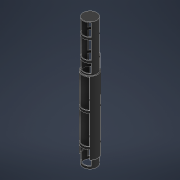
# Autodesk Inventor part: Test_Electronics_ Housing
Saved by Autodesk Inventor 2022 (Build 260153000, 153)
## iProperties
Created: 2024-05-09
Part Number: Test_Electronics_ Housing
Material: Generic
Document SubType Name: Modeling
Designer: jo_ki
Density: 1 g/cm^3
Appearance: Rubber - Black
Author: jo_ki
Autodesk Inventor part; units mm, degrees
ref_plane "YZ Plane" through (0, 0, 0) normal (1, 0, 0) x (0, 1, 0)
ref_plane "XZ Plane" through (0, 0, 0) normal (0, 1, 0) x (-1, 0, 0)
sketch "Sketch1" plane through (0, 0, 0) normal (0, 0, 1) x (1, 0, 0)
  line L0 (0, -222.05) -> (0, 149.3) projected
  line L1 (0, 0) -> (14, 0)
  line L2 (14, 0) -> (14, 96.25)
  line L3 (14, 96.25) -> (0, 96.25)
  line L4 (0, 96.25) -> (0, 0)
  line L5 (0, 0) -> (16, 0)
  line L6 (16, 0) -> (16, -150)
  line L7 (16, -150) -> (0, -150)
  line L8 (0, -150) -> (0, 0)
  line L9 (0, -150) -> (14, -150)
  line L10 (14, -150) -> (14, -169)
  line L11 (14, -169) -> (0, -169)
  line L12 (0, -169) -> (0, -150)
  line L13 (12.5, 94.75) -> (0, 94.75)
  line L14 (0, 94.75) -> (0, -1.5)
  line L15 (0, -1.5) -> (12.5, -1.5)
  line L16 (12.5, -1.5) -> (12.5, 94.75)
  line L17 (12.5, -167.5) -> (0, -167.5)
  line L18 (0, -167.5) -> (0, -148.5)
  line L19 (0, -148.5) -> (12.5, -148.5)
  line L20 (12.5, -148.5) -> (12.5, -167.5)
  line L21 (0, -1.5) -> (14.5, -1.5)
  line L22 (14.5, -1.5) -> (14.5, -148.5)
  line L23 (14.5, -148.5) -> (0, -148.5)
  line L24 (0, -148.5) -> (0, -1.5)
  line L25 (12.5, -167.5) -> (14, -167.5)
  point P0 (0, 96.25)
  point P1 (0, -169)
  point P2 (14, 0)
  point P3 (0, 94.75)
  point P4 (12.5, -1.5)
  point P5 (0, -167.5)
  dimension "d0" = 28
  dimension "d1" = 96.25
  dimension "d3" = 150
  dimension "d4" = 19
  dimension "d7" = 32
  dimension "d8" = 28
  dimension "d13" = 1.5
  dimension "d14" = 1.5
  dimension "d15" = 1.5
  dimension "d16" = 1.5
  dimension "d17" = 1.5
  dimension "d18" = 1.5
  constraints: 50 end point, 12 parallel, 7 perpendicular, 6 horizontal, 5 point on line, 2 collinear
  measures "d0" diameter of L2 L0
  measures "d1" distance of L1.end L2.end
  measures "d3" distance of L5.end L6.end
  measures "d4" distance of L9.end L10.end
  measures "d7" diameter of L6 L0
  measures "d8" diameter of L10 L0
  measures "d13" distance between parallel lines of L6 L22
  measures "d14" distance between parallel lines of L16 L2
  measures "d15" distance between parallel lines of L5 L21
  measures "d16" distance between parallel lines of L7 L23
  measures "d17" distance between parallel lines of L11 L17
  measures "d18" distance between parallel lines of L3 L13
revolve "Revolution1" add sketch "Sketch1" angle 360 about axis through (0, -10, 0) along (0, 1, 0) contours L20 L7 L10 L25 | L20 L23 L22 L21 L16 L1 L5 L6 L7 | L0 L3 L2 L1 L16 L13
sketch "Sketch2" plane through (0, 0, 0) normal (0, 1, 0) x (-1, 0, 0)
  circle A0 centre (0, 0) radius 16 projected
  line L0 (6, -12.6491) -> (6, -14.8324)
  circle A1 centre (0, 0) radius 16 projected
  line L1 (-6, -12.6491) -> (-6, -14.8324)
  line L2 (0, -22.4) -> (0, 22.4) projected
  circle A2 centre (0, 0) radius 14 projected
  point P0 (0, 16)
  point P1 (0, -16)
  dimension "d9" = 12
  constraints: 4 end point, 1 parallel, 1 point on circle, 1 vertical, 5 other
  measures "d9" distance between parallel lines of L1 L0
extrude "Extrusion1" [suppressed]
sketch "Sketch3" plane through (0, 0, 0) normal (0, 0, 1) x (1, 0, 0)
  line L0 (11, 94.75) -> (-11, 94.75)
  line L1 (-11, 94.75) -> (-11, -167.5)
  line L2 (-11, -167.5) -> (11, -167.5)
  line L3 (11, -167.5) -> (11, 94.75)
  line L4 (12.5, -167.5) -> (12.5, -148.5) projected
  line L5 (-12.5, -167.5) -> (-12.5, -148.5) projected
  line L6 (0, -219.95) -> (0, 147.2) projected
  line L7 (-12.5, -167.5) -> (12.5, -167.5) projected
  line L8 (-12.5, 94.75) -> (12.5, 94.75) projected
  line L9 (11, -131.5) -> (-11, -131.5)
  line L10 (-11, -131.5) -> (-11, -126.5)
  line L11 (-11, -126.5) -> (11, -126.5)
  line L12 (11, -126.5) -> (11, -131.5)
  line L13 (11, -66.5) -> (-11, -66.5)
  line L14 (-11, -66.5) -> (-11, -61.5)
  line L15 (-11, -61.5) -> (11, -61.5)
  line L16 (11, -61.5) -> (11, -66.5)
  line L17 (-12.5, -1.5) -> (-12.5, 94.75) projected
  line L18 (11, -1.5) -> (-12.5, -1.5)
  line L19 (-12.5, -1.5) -> (-12.5, 3.5)
  line L20 (-12.5, 3.5) -> (11, 3.5)
  line L21 (11, 3.5) -> (11, -1.5)
  line L22 (11, 63.5) -> (-11, 63.5)
  line L23 (-11, 63.5) -> (-11, 68.5)
  line L24 (-11, 68.5) -> (11, 68.5)
  line L25 (11, 68.5) -> (11, 63.5)
  line L26 (0, -126.5) -> (0, -66.5)
  line L27 (0, -61.5) -> (0, -1.5)
  line L28 (0, 3.5) -> (0, 63.5)
  line L29 (-12.5, -1.5) -> (12.5, -1.5) projected
  line L30 (-16, 0) -> (16, 0) projected
  line L31 (-16, -150) -> (16, -150) projected
  line L32 (-6, 0) -> (6, 0)
  line L33 (6, 0) -> (6, 27)
  line L34 (6, 27) -> (-6, 27)
  line L35 (-6, 27) -> (-6, 0)
  line L36 (11, 22) -> (-11, 22)
  line L37 (-11, 22) -> (-11, 27)
  line L38 (-11, 27) -> (11, 27)
  line L39 (11, 27) -> (11, 22)
  line L40 (-6, 22) -> (11, 22)
  line L41 (-12.5, -162.5) -> (12.5, -162.5)
  line L42 (12.5, -162.5) -> (12.5, -167.5)
  line L43 (12.5, -167.5) -> (-12.5, -167.5)
  line L44 (-12.5, -167.5) -> (-12.5, -162.5)
  point P0 (0, 0)
  point P1 (-11, -131.5)
  point P2 (-11, -66.5)
  point P3 (11, -126.5)
  point P4 (-11, -1.5)
  point P5 (11, -61.5)
  point P6 (-11, 63.5)
  point P7 (-11, 3.5)
  point P8 (11, 3.5)
  point P9 (11, 68.5)
  point P10 (-11, 22)
  point P11 (11, 27)
  point P12 (6, 22)
  point P13 (6, 3.5)
  point P14 (-6, 3.5)
  point P15 (-11, -162.5)
  point P16 (11, -162.5)
  dimension "d19" = 1.5
  dimension "d22" = 5
  dimension "d23" = 5
  dimension "d24" = 5
  dimension "d25" = 5
  dimension "d26" = 60
  dimension "d27" = 5
  dimension "d32" = 5
  constraints: 72 end point, 18 point on line, 16 parallel, 8 horizontal, 8 perpendicular, 7 collinear, 4 midpoint, 1 other
  measures "d19" distance between parallel lines of L3 L4
  measures "d22" distance between parallel lines of L11 L9
  measures "d23" distance between parallel lines of L13 L15
  measures "d24" distance between parallel lines of L18 L20
  measures "d25" distance between parallel lines of L22 L24
  measures "d26" distance of L27.start L27.end
  measures "d27" distance between parallel lines of L36 L38
  measures "d32" distance between parallel lines of L7 L41
extrude "Extrusion2" cut sketch "Sketch3" along normal through all both and the other way through all contours L3 L24 L6 L0 | L6 L24 L1 L0 | L3 L38 L34 L6 L22 | L6 L34 L38 L1 L22 | L3 L20 L33 L36 | L1 L36 L35 L20 | L36 L33 L20 L6 | L6 L20 L35 L36 | L18 L6 L15 L1 | L3 L15 L6 L18 | L13 L6 L11 L1 | L3 L11 L6 L13 | L9 L6 L31 L1 | L3 L31 L6 L9 | L31 L6 L41 L1 | L3 L41 L6 L31
sketch "Sketch4" plane through (0, 0, 0) normal (0, 1, 0) x (-1, 0, 0)
  circle A0 centre (0, 0) radius 16 projected
  circle A1 centre (0, 0) radius 12.5 projected
  line L0 (6, -10.9659) -> (6, -14.8324)
  line L1 (-6, -14.8324) -> (-6, -10.9659)
  line L2 (0, -22.4) -> (0, 22.4) projected
  dimension "d33" = 12
  constraints: 4 end point, 4 point on circle, 1 parallel, 1 vertical, 1 other
  measures "d33" distance between parallel lines of L1 L0
extrude "Extrusion3" add sketch "Sketch4" along normal blind 27 and the other way blind 5 contours A0 L2 A1 L0 | A0 L1 A1 L2 picked at (3.409, -13.2047) picked at (-3.409, -13.2047)
ref_plane "Work Plane1" through (0, -75, -16) normal (0, 0, 1) x (1, 0, 0)
sketch "Sketch5" plane through (0, -75, -16) normal (0, 0, 1) x (1, 0, 0)
  line L0 (-6, 73.5) -> (-11, 73.5) projected
  line L1 (-11, 73.5) -> (-11, 13.5) projected
  line L2 (-11, 13.5) -> (11, 13.5) projected
  line L3 (11, 13.5) -> (11, 73.5) projected
  line L4 (11, 73.5) -> (6, 73.5) projected
  line L5 (6, 70) -> (6, 73.5) projected
  line L6 (-6, 70) -> (6, 70) projected
  line L7 (-6, 73.5) -> (-6, 70) projected
  line L8 (6, 75) -> (-6, 75) projected
  line L9 (-6, 102) -> (-6, 75) projected
  line L10 (6, 102) -> (-6, 102) projected
  line L11 (6, 75) -> (6, 102) projected
  line L12 (11, -56.5) -> (11, -75) projected
  line L13 (11, -75) -> (11, -75) projected
  line L14 (11, -75) -> (11, -56.5) projected
  line L15 (11, -56.5) -> (-11, -56.5) projected
  line L16 (-11, -56.5) -> (-11, -75) projected
  line L17 (-11, -75) -> (-11, -75) projected
  line L18 (-11, -75) -> (-11, -56.5) projected
  line L19 (-11, -56.5) -> (11, -56.5) projected
  line L20 (-11, 73.5) -> (11, 73.5) projected
  line L21 (11, 73.5) -> (11, 13.5) projected
  line L22 (11, 13.5) -> (-11, 13.5) projected
  line L23 (-11, 13.5) -> (-11, 73.5) projected
  line L24 (-11, 8.5) -> (11, 8.5) projected
  line L25 (11, 8.5) -> (11, -51.5) projected
  line L26 (11, -51.5) -> (-11, -51.5) projected
  line L27 (-11, -51.5) -> (-11, 8.5) projected
  line L28 (11, 8.5) -> (-11, 8.5) projected
  line L29 (-11, 8.5) -> (-11, -51.5) projected
  line L30 (-11, -51.5) -> (11, -51.5) projected
  line L31 (11, -51.5) -> (11, 8.5) projected
  line L32 (-6, 70) -> (6, 70) projected
  line L33 (-6, 70) -> (-6, 102)
  line L34 (-6, 102) -> (-6, 75) projected
  line L35 (-6, 86) -> (6, 86)
  line L36 (0, -145.25) -> (0, 224) projected
  point P0 (0, 75)
  point P1 (0, 96)
  point P2 (0, 76)
  point P3 (0, 86)
  dimension "d38" = 20
  constraints: 5 point on line, 4 end point, 2 midpoint, 2 perpendicular, 1 symmetric about line
  measures "d38" distance of point (0, 76) point (0, 96)
hole "Hole1" at (0, 21, -16) at (0, 1, -16) direction (0, 0, 1) diameter 3.5 depth 10
hole "Hole2" at (0, 11, -16) direction (0, 0, 1) diameter 5 depth 1.25
equation "\"d14\" = d13"
equation "\"d15\" = d13"
equation "\"d16\" = d13"
equation "\"d17\" = d13"
equation "\"d18\" = d13"
equation "\"d23\" = d22"
equation "\"d24\" = d22"
equation "\"d25\" = d23"
equation "\"d27\" = d24"
body "Solid1"
